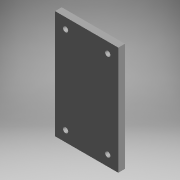
# Autodesk Inventor part: yCarraige
Saved by Autodesk Inventor 2019 (Build 230136000, 136)
## iProperties
Created: 2019-05-08
Part Number: yCarraige
Material: Generic
Document SubType Name: Modeling
Designer: Alex Jones
Density: 1 g/cm^3
Appearance: Default
Author: Alex Jones
Autodesk Inventor part; units mm, degrees
ref_plane "YZ Plane" through (0, 0, 0) normal (1, 0, 0) x (0, 1, 0)
ref_plane "XZ Plane" through (0, 0, 0) normal (0, 1, 0) x (-1, 0, 0)
ref_plane "XY Plane" through (0, 0, 0) normal (0, 0, 1) x (1, 0, 0)
sketch "Sketch1" plane through (0, 0, 0) normal (0, 0, 1) x (1, 0, 0)
  circle A0 centre (-610.9072, 17.8) radius 2.5 projected
  circle A1 centre (-610.9072, 17.8) radius 9.9 construction
  circle A2 centre (-650.9072, 17.8) radius 2.5 projected
  circle A3 centre (-650.9072, 17.8) radius 9.9 construction
  circle A4 centre (-610.9071, -65) radius 2.5 projected
  circle A5 centre (-610.9071, -65) radius 9.9 construction
  circle A6 centre (-650.9072, -65) radius 2.5 projected
  circle A7 centre (-650.9072, -65) radius 9.9 construction
  line L0 (-610.9071, -65) -> (-650.9072, -65) construction
  line L1 (-650.9072, -65) -> (-650.9072, 17.8) construction
  line L2 (-650.9072, 17.8) -> (-610.9071, 17.8) construction
  line L3 (-610.9071, 17.8) -> (-610.9071, -65) construction
  line L4 (-660.9072, -75) -> (-600.9071, -75)
  line L5 (-600.9071, -75) -> (-600.9071, 27.8)
  line L6 (-600.9071, 27.8) -> (-660.9072, 27.8)
  line L7 (-660.9072, 27.8) -> (-660.9072, -75)
  point P0 (0, 0)
  dimension "d0" = 10
  constraints: 16 end point, 4 parallel, 2 perpendicular, 1 horizontal, 3 other
  measures "d0" distance between parallel lines of L0 L4
extrude "Extrusion1" add sketch "Sketch1" along normal blind 6.35
body "Solid1"
